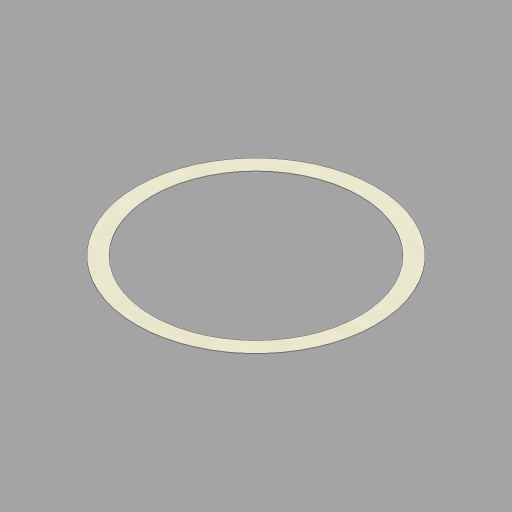
# Autodesk Inventor part: TorsionOscillator-IsolationRing
Saved by Autodesk Inventor 2024 (Build 280153020, 153B)
## iProperties
Created: 2023-08-21
Part Number: TorsionOscillator-IsolationRing
Material: Paper
Document SubType Name: Modeling
Designer: schanen
Density: 0.93 g/cm^3
Appearance: Cardboard - Chipboard
Author: schanen
Autodesk Inventor part; units mm, degrees
ref_plane "YZ Plane" through (0, 0, 0) normal (1, 0, 0) x (0, 1, 0)
ref_plane "XZ Plane" through (0, 0, 0) normal (0, 1, 0) x (-1, 0, 0)
ref_plane "XY Plane" through (0, 0, 0) normal (0, 0, 1) x (1, 0, 0)
sketch "Sketch1" plane through (0, 0, 0) normal (0, 0, 1) x (1, 0, 0)
  line L0 (-20, 0) -> (-23, 0)
  line L1 (-23, 0) -> (-23, 0.1)
  line L2 (-23, 0.1) -> (-20, 0.1)
  line L3 (-20, 0.1) -> (-20, 0)
  line L4 (0, -0.02) -> (0, 0.12) projected
  point P0 (0, 0)
  dimension "d0" = 20
  dimension "d1" = 23
  dimension "d2" = 0.1
  constraints: 8 end point, 2 parallel, 1 horizontal, 1 perpendicular
  measures "d0" distance of point (0, 0) L0.start
  measures "d1" distance of point (0, 0) L0.end
  measures "d2" distance of L0.end L1.end
revolve "Revolution1" add sketch "Sketch1" angle 360 about axis through (0, -10, 0) along (0, 1, 0)
body "Solid1"
